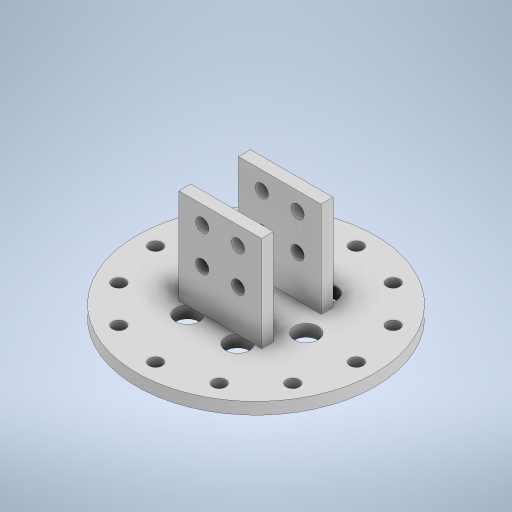
# Autodesk Inventor part: Base
Saved by Autodesk Inventor 2023 (Build 270158000, 158)
## iProperties
Created: 2023-12-18
Part Number: Base
Material: Generic
Document SubType Name: Modeling
Designer: Mustapha
Density: 1 g/cm^3
Appearance: Default
Author: Mustapha
Autodesk Inventor part; units mm, degrees
ref_plane "YZ Plane" through (0, 0, 0) normal (1, 0, 0) x (0, 1, 0)
ref_plane "XZ Plane" through (0, 0, 0) normal (0, 1, 0) x (-1, 0, 0)
ref_plane "XY Plane" through (0, 0, 0) normal (0, 0, 1) x (1, 0, 0)
sketch "Sketch1" plane through (0, 0, 0) normal (0, 1, 0) x (-1, 0, 0)
  circle A0 centre (0, 0) radius 50
  circle A1 centre (42.1286, 0) radius 2.75
  circle A2 centre (36.4845, -21.0643) radius 2.75
  circle A3 centre (21.0643, -36.4845) radius 2.75
  circle A4 centre (0, -42.1286) radius 2.75
  circle A5 centre (-21.0643, -36.4845) radius 2.75
  circle A6 centre (-36.4845, -21.0643) radius 2.75
  circle A7 centre (-42.1286, 0) radius 2.75
  circle A8 centre (-36.4845, 21.0643) radius 2.75
  circle A9 centre (-21.0643, 36.4845) radius 2.75
  circle A10 centre (0, 42.1286) radius 2.75
  circle A11 centre (21.0643, 36.4845) radius 2.75
  circle A12 centre (36.4845, 21.0643) radius 2.75
  circle A13 centre (21.0643, 0) radius 5
  circle A14 centre (10.5322, 18.2422) radius 5
  circle A15 centre (-10.5322, 18.2422) radius 5
  circle A16 centre (-21.0643, 0) radius 5
  circle A17 centre (-10.5322, -18.2422) radius 5
  circle A18 centre (10.5322, -18.2422) radius 5
  dimension "d0" = 100
  dimension "d1" = 5.5
  dimension "d4" = 360
  dimension "d6" = 10
  dimension "d9" = 360
  constraints: 19 centre point, 3 coincident, 48 other
  measures "d0" diameter of A0
  measures "d1" diameter of A1
  measures "d6" diameter of A13
extrude "Extrusion1" add sketch "Sketch1" along normal blind 5
sketch "Sketch2" plane through (0, 5, 0) normal (0, 1, 0) x (1, 0, 0)
  line L0 (0, 0) -> (-49.6447, 0)
  line L1 (0, 0) -> (0, 30.1523)
  line L2 (-17.3205, -10) -> (17.3205, -10)
  line L3 (17.3205, -10) -> (17.3205, -15)
  line L4 (17.3205, -15) -> (-17.3205, -15)
  line L5 (-17.3205, -15) -> (-17.3205, -10)
  line L6 (-17.3205, -10) -> (17.3205, -15) construction
  line L7 (17.3205, -10) -> (-17.3205, -15) construction
  line L8 (-17.3205, 10) -> (17.3205, 10)
  line L9 (17.3205, 10) -> (17.3205, 15)
  line L10 (17.3205, 15) -> (-17.3205, 15)
  line L11 (-17.3205, 15) -> (-17.3205, 10)
  line L12 (-17.3205, 10) -> (17.3205, 15) construction
  line L13 (17.3205, 10) -> (-17.3205, 15) construction
  point P0 (0, -12.5)
  point P1 (0, 12.5)
  dimension "d13" = 20
  dimension "d14" = 34.641
  dimension "d17" = 0
  dimension "d18" = 5
  constraints: 28 end point, 5 symmetric about line, 2 horizontal, 2 midpoint, 2 parallel, 1 perpendicular, 1 vertical
  measures "d13" diameter of L2 L0
  measures "d14" distance of L3.end L4.end
  measures "d17" horizontal distance of L0.start point (0, -12.5)
  measures "d18" distance between parallel lines of L2 L4
extrude "Extrusion2" add sketch "Sketch2" along normal blind 40
sketch "Sketch4" plane through (-17.3205, 5, 15) normal (0, 0, 1) x (1, 0, 0)
  line L0 (24.8205, 32.5) -> (9.8205, 32.5)
  line L1 (9.8205, 32.5) -> (9.8205, 17.5)
  line L2 (9.8205, 17.5) -> (24.8205, 17.5)
  line L3 (24.8205, 17.5) -> (24.8205, 32.5)
  line L4 (24.8205, 32.5) -> (9.8205, 17.5) construction
  line L5 (9.8205, 32.5) -> (24.8205, 17.5) construction
  line L6 (34.641, 0) -> (34.641, 40) projected
  line L7 (0, 40) -> (34.641, 40) projected
  circle A0 centre (9.8205, 32.5) radius 2.75
  circle A1 centre (24.8205, 32.5) radius 2.75
  circle A2 centre (24.8205, 17.5) radius 2.75
  circle A3 centre (9.8205, 17.5) radius 2.75
  point P0 (17.3205, -5)
  point P1 (17.3205, 25)
  dimension "d23" = 15
  dimension "d24" = 17.3205
  dimension "d25" = 15
  dimension "d26" = 15
  dimension "d27" = 5.5
  dimension "d28" = 5.5
  dimension "d29" = 5.5
  dimension "d30" = 5.5
  constraints: 12 end point, 4 centre point, 4 coincident, 2 midpoint, 2 parallel, 1 horizontal, 1 perpendicular
  measures "d23" distance of L0.start L0.end
  measures "d24" distance from line of L6 point (17.321, 25)
  measures "d25" distance from line of point (17.321, 25) L7
  measures "d26" distance between parallel lines of L2 L0
  measures "d27" diameter of A0
  measures "d28" diameter of A1
  measures "d29" diameter of A2
  measures "d30" diameter of A3
extrude "Extrusion3" cut sketch "Sketch4" against normal blind 80 contours A0 L1 L0 | L0 L1 A0 | A1 L3 L0 | L0 L3 A1 | A3 L2 L1 | L1 L2 A3 | A2 L2 L3 | L3 L2 A2
body "Solid1"
